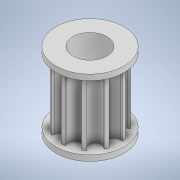
# Autodesk Inventor part: Pièce_moteur_courroie_test_6
Saved by Autodesk Inventor 2020.1 (Build 241239000, 239)
## iProperties
Created: 2019-07-26
Part Number: Pièce_moteur_courroie_test_6
Material: Générique
Document SubType Name: Modeling
Designer: marlo
Density: 1 g/cm^3
Appearance: Par défaut
Author: marlo
Autodesk Inventor part; units mm, degrees
ref_plane "YZ Plane" through (0, 0, 0) normal (1, 0, 0) x (0, 1, 0)
ref_plane "XZ Plane" through (0, 0, 0) normal (0, 1, 0) x (-1, 0, 0)
ref_plane "XY Plane" through (0, 0, 0) normal (0, 0, 1) x (1, 0, 0)
sketch "Esquisse2" plane through (0, 0, 0) normal (0, 1, 0) x (-1, 0, 0)
  circle A0 centre (0, 0) radius 7.6
  dimension "d0" = 15.2
  constraints: 1 centre point, 1 coincident
  measures "d0" diameter of A0
extrude "Extrusion1" add sketch "Esquisse2" along normal blind 17
sketch "Esquisse4" plane through (0, 17, 0) normal (0, 1, 0) x (1, 0, 0)
  circle A0 centre (0, 0) radius 7.6 projected
  circle A1 centre (0, 0) radius 7.6 projected
  arc A2 (-3.2, -6.8935) -> (0, -7.6) centre (0, 0) ccw
  line L0 (-0.0062, -0.0113) -> (-4.6214, -8.4012)
  line L1 (0, -6.3735) -> (0, 5.2233) construction
  line L2 (-3.2, -6.8935) -> (0, -7.6) construction
  line L3 (-3.2, -6.8935) -> (-3.0675, -6.2935)
  line L4 (0, -7.6) -> (0.1325, -7)
  arc A3 (0.1325, -7) -> (-3.0675, -6.2935) centre (-1.4675, -6.6467) ccw
  line L5 (-3.0675, -6.2935) -> (0.1325, -7) construction
  arc A4 (-6.419, -4.069) -> (-4.109, -6.3935) centre (0, 0) ccw
  line L6 (-4.109, -6.3935) -> (-6.419, -4.069) construction
  line L7 (-4.109, -6.3935) -> (-3.6731, -5.9603)
  line L8 (-6.419, -4.069) -> (-5.9831, -3.6359)
  arc A5 (-3.6731, -5.9603) -> (-5.9831, -3.6359) centre (-4.8281, -4.7981) ccw
  line L9 (-3.6731, -5.9603) -> (-5.9831, -3.6359) construction
  line L10 (-4.109, -6.3935) -> (-3.2, -6.8935) construction
  line L11 (0, 0) -> (-8.9658, -4.8594)
  arc A6 (-6.3677, 4.1487) -> (-7.5226, 1.0819) centre (0, 0) ccw
  line L12 (-7.5226, 1.0819) -> (-6.3677, 4.1487) construction
  line L13 (-7.5226, 1.0819) -> (-6.9476, 0.8653)
  line L14 (-6.3677, 4.1487) -> (-5.7927, 3.9322)
  arc A7 (-6.9476, 0.8653) -> (-5.7927, 3.9322) centre (-6.3701, 2.3988) ccw
  line L15 (-6.9476, 0.8653) -> (-5.7927, 3.9322) construction
  arc A8 (-7.5999, 0.0474) -> (-6.9133, -3.157) centre (0, 0) ccw
  line L16 (-7.5999, 0.0474) -> (-6.9133, -3.157) construction
  line L17 (-7.5999, 0.0474) -> (-6.999, 0.1761)
  line L18 (-6.9133, -3.157) -> (-6.3125, -3.0282)
  arc A9 (-6.3125, -3.0282) -> (-6.999, 0.1761) centre (-6.6558, -1.4261) ccw
  line L19 (-6.999, 0.1761) -> (-6.3125, -3.0282) construction
  line L20 (-7.5999, 0.0474) -> (-7.5226, 1.0819) construction
  line L21 (-6.9133, -3.157) -> (-6.419, -4.069) construction
  line L22 (0, 0) -> (-6.7758, 5.1057)
  arc A10 (7.3055, 2.0952) -> (5.7441, 4.9764) centre (0, 0) ccw
  line L23 (5.7441, 4.9764) -> (7.3055, 2.0952) construction
  line L24 (5.7441, 4.9764) -> (5.2039, 4.6837)
  line L25 (7.3055, 2.0952) -> (6.7653, 1.8025)
  arc A11 (5.2039, 4.6837) -> (6.7653, 1.8025) centre (5.9846, 3.2431) ccw
  line L26 (5.2039, 4.6837) -> (6.7653, 1.8025) construction
  arc A12 (5.0129, 5.7123) -> (2.1417, 7.292) centre (0, 0) ccw
  line L27 (5.0129, 5.7123) -> (2.1417, 7.292) construction
  line L28 (5.0129, 5.7123) -> (4.7167, 5.174)
  line L29 (2.1417, 7.292) -> (1.8455, 6.7536)
  arc A13 (1.8455, 6.7536) -> (4.7167, 5.174) centre (3.2811, 5.9638) ccw
  line L30 (4.7167, 5.174) -> (1.8455, 6.7536) construction
  line L31 (5.0129, 5.7123) -> (5.7441, 4.9764) construction
  line L32 (-3.1138, 6.9328) -> (-2.7472, 6.4398)
  arc A14 (-5.3768, 4.4842) -> (-2.7472, 6.4398) centre (-4.062, 5.462) ccw
  line L33 (-2.7472, 6.4398) -> (-5.3768, 4.4842) construction
  line L34 (-3.1138, 6.9328) -> (-5.7434, 4.9772) construction
  arc A15 (-3.1138, 6.9328) -> (-5.7434, 4.9772) centre (0, 0) ccw
  line L35 (-5.7434, 4.9772) -> (-5.3768, 4.4842)
  line L36 (-2.1407, 7.2923) -> (-3.1138, 6.9328) construction
  line L37 (-2.1407, 7.2923) -> (-2.0988, 6.6793)
  line L38 (-2.0988, 6.6793) -> (1.1706, 6.9027) construction
  line L39 (-2.1407, 7.2923) -> (1.1287, 7.5157) construction
  arc A16 (1.1287, 7.5157) -> (-2.1407, 7.2923) centre (0, 0) ccw
  arc A17 (-2.0988, 6.6793) -> (1.1706, 6.9027) centre (-0.4641, 6.791) ccw
  line L40 (1.1287, 7.5157) -> (1.1706, 6.9027)
  line L41 (1.1287, 7.5157) -> (2.1417, 7.292) construction
  line L42 (-6.3677, 4.1487) -> (-5.7434, 4.9772) construction
  line L43 (0, 0) -> (10.678, -14.3583) construction
  arc A18 (7.2785, -2.1871) -> (7.5228, 1.0808) centre (0, 0) ccw
  line L44 (7.5228, 1.0808) -> (7.2785, -2.1871) construction
  line L45 (7.5228, 1.0808) -> (6.91, 1.1266)
  line L46 (7.2785, -2.1871) -> (6.6658, -2.1413)
  arc A19 (6.91, 1.1266) -> (6.6658, -2.1413) centre (6.7879, -0.5073) ccw
  line L47 (6.91, 1.1266) -> (6.6658, -2.1413) construction
  line L48 (7.3055, 2.0952) -> (7.5228, 1.0808) construction
  line L49 (7.2785, -2.1871) -> (0, -7.6) construction
  line L50 (0, 0) -> (10.2791, -3.8716)
  line L51 (1.0339, -7.5293) -> (0.8211, -6.9529)
  arc A20 (3.8952, -5.8176) -> (0.8211, -6.9529) centre (2.3581, -6.3853) ccw
  arc A21 (1.0339, -7.5293) -> (4.1081, -6.394) centre (0, 0) ccw
  line L52 (4.1081, -6.394) -> (3.8952, -5.8176)
  line L53 (0.8211, -6.9529) -> (3.8952, -5.8176) construction
  line L54 (4.9405, -5.775) -> (4.4498, -5.4052)
  arc A22 (6.4221, -2.7881) -> (4.4498, -5.4052) centre (5.436, -4.0967) ccw
  line L55 (4.4498, -5.4052) -> (6.4221, -2.7881) construction
  line L56 (4.9405, -5.775) -> (6.9128, -3.1579) construction
  arc A23 (4.9405, -5.775) -> (6.9128, -3.1579) centre (0, 0) ccw
  line L57 (6.9128, -3.1579) -> (6.4221, -2.7881)
  line L58 (7.2785, -2.1871) -> (6.9128, -3.1579) construction
  point P0 (-7.5999, 0.0474)
  point P1 (-6.9133, -3.157)
  point P2 (-6.3677, 4.1487)
  point P3 (-7.5226, 1.0819)
  point P4 (-3.1138, 6.9328)
  point P5 (-5.7434, 4.9772)
  point P6 (1.1287, 7.5157)
  point P7 (-2.1407, 7.2923)
  point P8 (5.0129, 5.7123)
  point P9 (2.1417, 7.292)
  point P10 (7.3055, 2.0952)
  point P11 (5.7441, 4.9764)
  point P12 (-3.2, -6.8935)
  point P13 (0, -7.6)
  point P14 (-6.419, -4.069)
  point P15 (-4.109, -6.3935)
  point P16 (7.2785, -2.1871)
  point P17 (7.5228, 1.0808)
  point P18 (4.9405, -5.775)
  point P19 (4.9405, -5.775)
  point P20 (6.9128, -3.1579)
  point P21 (1.0339, -7.5293)
  point P22 (4.1081, -6.394)
  dimension "d14" = 3.2
  dimension "d28" = 0.6
  dimension "d30" = 0.5
  constraints: 118 end point, 51 symmetric about line, 50 point on circle, 22 centre point, 5 equal length, 5 point on line, 3 perpendicular, 1 coincident, 1 midpoint, 1 vertical, 20 other
  measures "d14" horizontal distance of L2.start L2.end
  measures "d28" vertical distance of L2.start L3.end
  measures "d30" vertical distance of L6.start L2.start
extrude "Extrusion6" cut sketch "Esquisse4" against normal through all contours A0 L46 A19 L45 | L25 A11 L24 A0 | A0 L54 A22 L57 | L28 A13 L29 A0 | A0 L51 A20 L52 | A0 L17 A9 L18 | L8 A5 L7 A0 | A0 L32 A14 L35 | L14 A7 L13 A0 | L40 A17 L37 A0 | A0 L3 A3 L4
sketch "Esquisse6" plane through (0, 17, 0) normal (0, 1, 0) x (1, 0, 0)
  circle A0 centre (0, 0) radius 9
  dimension "d19" = 18
  constraints: 1 centre point, 1 coincident
  measures "d19" diameter of A0
extrude "Extrusion3" add sketch "Esquisse6" along normal blind 1.5
sketch "Esquisse7" plane through (0, 0, 0) normal (0, -1, 0) x (1, 0, 0)
  circle A0 centre (0, 0) radius 9
  dimension "d34" = 18
  constraints: 1 centre point, 1 coincident
  measures "d34" diameter of A0
extrude "Extrusion4" add sketch "Esquisse7" along normal blind 1.5
sketch "Esquisse8" plane through (0, 18.5, 0) normal (0, 1, 0) x (1, 0, 0)
  circle A0 centre (0, 0) radius 4.5
  dimension "d24" = 9
  constraints: 1 centre point, 1 coincident
  measures "d24" diameter of A0
extrude "Extrusion5" cut sketch "Esquisse8" against normal through all
